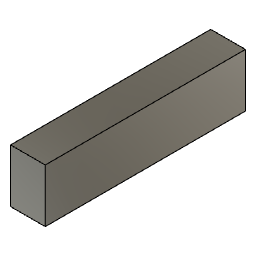
스위치 홈 (Autodesk Fusion 360 design; units mm, degrees)
Autodesk Fusion 360 part; units mm, degrees
note: some values were not read from the file. Set by a fixed rule: which face or edge a step refers to.
sketch "스케치1" plane through (0, 0, 0) normal (0, 0, 1) x (1, 0, 0)
  line L0 (-5, 0) -> (15, 0)
  line L1 (15, 0) -> (15, -30)
  line L2 (15, -30) -> (-5, -30)
  line L3 (-5, -30) -> (-5, 0)
  line L4 (-5, 0) -> (15, 0)
  line L5 (15, 0) -> (15, 50)
  line L6 (15, 50) -> (-5, 50)
  line L7 (-5, 50) -> (-5, 0)
  line L8 (-4, 50) -> (-4, 45)
  line L9 (-4, 45) -> (-4, 0)
  line L10 (14, 50) -> (14, 0)
  line L11 (-5, -30) -> (-5, 0)
  line L12 (15, 0) -> (15, -30)
  line L13 (15, -30) -> (-5, -30)
  line L14 (15, 50) -> (-5, 50)
  line L15 (-5, 0) -> (15, 0)
  line L16 (14, 50) -> (14, 0)
  line L17 (15, 0) -> (15, 50)
  line L18 (-5, 0) -> (15, 0)
  line L19 (-5, 50) -> (-5, 0)
  line L20 (-5, 0) -> (-5, 30)
  line L21 (15, 30) -> (-5, 30)
  line L22 (-5, 0) -> (-5, 40)
  line L23 (-5, 40) -> (15, 40)
  line L24 (-5, -10) -> (15, -10)
  line L25 (125, 0) -> (125, 30)
  line L26 (125, 0) -> (125, 40)
  line L27 (125, 40) -> (145, 40)
  line L28 (125, 50) -> (125, 0)
  line L29 (125, -10) -> (145, -10)
  line L30 (145, 0) -> (145, -30)
  line L31 (144, 50) -> (144, 0)
  line L32 (126, 45) -> (126, 0)
  line L33 (144, 50) -> (144, 0)
  line L34 (125, -30) -> (125, 0)
  line L35 (145, 50) -> (125, 50)
  line L36 (145, -30) -> (125, -30)
  line L37 (125, -30) -> (125, 0)
  line L38 (125, 0) -> (145, 0)
  line L39 (125, 0) -> (145, 0)
  line L40 (145, -30) -> (125, -30)
  line L41 (125, 0) -> (145, 0)
  line L42 (145, 0) -> (145, -30)
  line L43 (145, 30) -> (125, 30)
  line L44 (125, 0) -> (145, 0)
  line L45 (145, 0) -> (145, 50)
  line L46 (125, 50) -> (125, 0)
  line L47 (145, 50) -> (125, 50)
  line L48 (145, 0) -> (145, 50)
  line L49 (126, 50) -> (126, 45)
  point P0 (130, 0)
  point P1 (130, 0)
  dimension "d1" = 30
  dimension "d2" = 20
  dimension "d3" = 50
  dimension "d6" = 1
  dimension "d7" = 1
  dimension "d8" = 30
  dimension "d9" = 20
  dimension "d10" = 50
  dimension "d12" = 1
  dimension "d23" = 30
  dimension "d24" = 40
  dimension "d25" = 10
  dimension "d26" = 30
  dimension "d27" = 20
  dimension "d28" = 50
  dimension "d29" = 1
  dimension "d30" = 1
  dimension "d31" = 30
  dimension "d32" = 20
  dimension "d33" = 50
  dimension "d34" = 1
  dimension "d35" = 30
  dimension "d36" = 40
  dimension "d37" = 10
  constraint horizontal L0
  constraint vertical L1
  constraint horizontal L2
  constraint vertical L3
  constraint horizontal L4
  constraint vertical L5
  constraint horizontal L6
  constraint vertical L7
  constraint coincident L6 L8.start
  constraint perpendicular L6 L8
  constraint coincident L0 L9.end
  constraint perpendicular L0 L9
  constraint coincident L6 L10.start
  constraint coincident L0 L10.end
  constraint perpendicular L6 L10
  constraint horizontal L15
  constraint vertical L12
  constraint horizontal L13
  constraint vertical L11
  constraint horizontal L18
  constraint vertical L17
  constraint horizontal L14
  constraint vertical L19
  constraint coincident L10.start L14
  constraint coincident L10.end L15
  constraint perpendicular L14 L16
  constraint coincident L19 L20.end
  constraint perpendicular L4 L20
  constraint coincident L5 L21.start
  constraint perpendicular L7 L21
  constraint perpendicular L21 L22
  constraint coincident L17 L23.end
  constraint perpendicular L17 L23
  constraint coincident L1 L24.end
  constraint perpendicular L1 L24
  constraint horizontal L41
  constraint vertical L42
  constraint horizontal L36
  constraint vertical L34
  constraint horizontal L38
  constraint vertical L48
  constraint horizontal L47
  constraint vertical L28
  constraint coincident L49.start L47
  constraint perpendicular L47 L49
  constraint coincident L32.end L41
  constraint perpendicular L32 L41
  constraint coincident L31.start L47
  constraint coincident L31.end L41
  constraint perpendicular L31 L47
  constraint horizontal L44
  constraint vertical L30
  constraint horizontal L40
  constraint vertical L37
  constraint horizontal L39
  constraint vertical L45
  constraint horizontal L35
  constraint vertical L46
  constraint coincident L31.start L35
  constraint coincident L31.end L44
  constraint perpendicular L33 L35
  constraint coincident L25.end L46
  constraint perpendicular L25 L38
  constraint coincident L43.start L48
  constraint perpendicular L28 L43
  constraint perpendicular L26 L43
  constraint coincident L27.end L45
  constraint perpendicular L27 L45
  constraint coincident L29.end L42
  constraint perpendicular L29 L42
  measures "d1" distance of L0.end L1.end
  measures "d2" distance of L1.end L2.end
  measures "d3" distance of L0.end L5.end
  measures "d6" distance of L7 L9
  measures "d7" distance of L5 L10
  measures "d8" distance of L0.end L1.end
  measures "d9" distance of L1.end L2.end
  measures "d10" distance of L5.end L0.end
  measures "d12" distance of L16 L17
  measures "d23" distance of L15 L21
  measures "d24" distance of L0.start L22.end
  measures "d25" distance of L0.start L24.start
  measures "d26" distance of L30.start L30.end
  measures "d27" distance of L30.end L34.start
  measures "d28" distance of L35.start L30.start
  measures "d29" distance of L28 L32
  measures "d30" distance of L31 L48
  measures "d31" distance of L30.end L30.start
  measures "d32" distance of L34.start L30.end
  measures "d33" distance of L30.start L35.start
  measures "d34" distance of L33 L45
  measures "d35" distance of L43 L44
  measures "d36" distance of L25.start L26.end
  measures "d37" distance of L25.start L29.start
extrude "돌출1" add sketch "스케치1" along normal blind 30 contours L1 L2 L3 L11 L12 L13 L24 makes body 1
extrude "돌출2" add sketch "스케치1" along normal blind 30 contours L0 L1 L3 L4 L11 L12 L15 L18 L24 bodies 1
extrude "돌출3" add sketch "스케치1" along normal blind 30 contours L0 L4 L5 L10 L15 L16 L17 L18 L21 bodies 1
extrude "돌출4" add sketch "스케치1" along normal blind 30 contours L0 L4 L7 L9 L15 L18 L19 L20 L21 L22 bodies 1
extrude "돌출5" add sketch "스케치1" along normal blind 30 separate body contours L29 L30 L34 L36 L37 L40 L42 makes body 2
extrude "돌출6" add sketch "스케치1" along normal blind 30 contours L29 L30 L34 L37 L38 L39 L41 L42 L44 bodies 2
extrude "돌출7" add sketch "스케치1" along normal blind 30 contours L25 L26 L28 L32 L38 L39 L41 L43 L44 L46 | L31 L33 L38 L39 L41 L43 L44 L45 L48 bodies 2
extrude "돌출8" add sketch "스케치1" along normal blind 30 contours L7 L9 L19 L21 L22 L23 | L6 L7 L8 L9 L14 L19 L23 | L5 L10 L16 L17 L21 L23 | L5 L6 L10 L14 L16 L17 L23 | L26 L27 L28 L32 L43 L46 | L27 L28 L32 L35 L46 L47 L49 | L27 L31 L33 L43 L45 L48 | L27 L31 L33 L35 L45 L47 L48 bodies 1 2
extrude "돌출9" cut 2 faces at (138, -20, 30) (8, -20, 30) along direction (0, 0, -1) blind 10 on bodies 1 2 bodies 1 2
sketch "스케치2" plane through (0, 0, 0) normal (0, 1, 0) x (-1, 0, 0)
  line L0 (4, 20) -> (-14, 20)
  line L1 (-14, 20) -> (-14, 0)
  line L2 (-14, 0) -> (4, 0)
  line L3 (4, 0) -> (4, 20)
  line L4 (-126, 20) -> (-144, 20)
  line L5 (-144, 20) -> (-144, 0)
  line L6 (-144, 0) -> (-126, 0)
  line L7 (-126, 0) -> (-126, 20)
  line L8 (-138, 17) -> (-128, 17)
  line L9 (-128, 17) -> (-128, 3)
  line L10 (-128, 3) -> (-138, 3)
  line L11 (-138, 3) -> (-138, 17)
  line L12 (-12, 17) -> (-2, 17)
  line L13 (-2, 17) -> (-2, 3)
  line L14 (-2, 3) -> (-12, 3)
  line L15 (-12, 3) -> (-12, 17)
  dimension "d56" = 2
  dimension "d57" = 2
  dimension "d58" = 10
  dimension "d59" = 10
  constraint horizontal L8
  constraint vertical L9
  constraint horizontal L10
  constraint vertical L11
  constraint horizontal L12
  constraint vertical L13
  constraint horizontal L14
  constraint vertical L15
  measures "d56" distance of L7 L9
  measures "d57" distance of L1 L15
  measures "d58" distance of L9 L11
  measures "d59" distance of L13 L15
extrude "돌출10" cut sketch "스케치2" against normal blind 10 contours L8 L9 L10 L11 | L12 L13 L14 L15 bodies 1 2
extrude "돌출11" cut 2 faces at (131.3333, -10, 7.6667) (8.6667, -10, 12.3333) along direction (0, -1, 0) blind 15 on bodies 1 2 bodies 1 2
extrude "돌출12" add sketch "스케치1" along normal blind 20 contours L27 L31 L32 L33 L35 L47 L49 bodies 2
extrude "돌출13" cut 1 faces at (131.3333, -25, 7.6667) along direction (0, 1, 0) blind 75 on bodies 2 bodies 2
move_face "면 간격띄우기1" offset -2 2 faces at (134.6667, 43.3333, 17) (131.3333, 43.3333, 3) on bodies 2
extrude "돌출14" add 1 faces at (134.6667, -25, 12.3333) along direction (0, 1, 0) blind 25 on bodies 2 bodies 2
extrude "돌출15" add sketch "스케치1" along normal blind 20 contours L6 L8 L9 L10 L14 L16 L23 bodies 1
move_face "면 간격띄우기2" offset -4 1 faces at (2, -8.3333, 12.3333) on bodies 1
sketch "스케치3" plane through (0, 0, 20) normal (0, 0, 1) x (-1, 0, 0)
  line L0 (-14, -40) -> (-14, 0)
  line L1 (-14, 0) -> (4, 0)
  line L2 (4, 0) -> (4, -40)
  line L3 (4, -40) -> (-14, -40)
  line L4 (-15, -50) -> (5, -50)
  line L5 (5, -50) -> (5, 30)
  line L6 (5, 30) -> (-15, 30)
  line L7 (-15, 30) -> (-15, -50)
  line L8 (-14, 26.9594) -> (4, 26.9594)
  line L9 (4, 26.9594) -> (4, 21.9594)
  line L10 (4, 21.9594) -> (-14, 21.9594)
  line L11 (-14, 21.9594) -> (-14, 26.9594)
  dimension "d74" = 5
  constraint horizontal L8
  constraint vertical L9
  constraint horizontal L10
  constraint vertical L11
  measures "d74" distance of L8.start L10.end
extrude "돌출16" cut sketch "스케치3" against normal blind 18 contours L8 L9 L10 L11 bodies 1
extrude "돌출17" add 1 faces at (8, -25.2927, 2) along direction (0, 0, 1) blind 1 on bodies 1 bodies 1
move_face "면 간격띄우기3" offset 5 1 faces at (138, 46.6667, 7) on bodies 2
move_face "면 간격띄우기4" offset 2 2 faces at (12, -7.3198, 7.6667) (-2, -7.3198, 12.3333) on bodies 1
extrude "돌출18" add sketch "스케치1" along normal blind 2 from surface at 18 contours L0 L4 L9 L10 L15 L16 L18 L21 | L9 L10 L16 L21 L23 bodies 1
extrude "돌출19" add sketch "스케치1" along normal blind 3 from surface at 17 contours L31 L32 L33 L38 L39 L41 L43 L44 | L27 L31 L32 L33 L43 bodies 2
extrude "돌출20" add sketch "스케치1" against normal blind 1 from surface at 17 separate body contours L0 L4 L9 L10 L15 L16 L18 L21 | L9 L10 L16 L21 L23 makes body 3
extrude "돌출21" add 1 faces at (134.3333, 13.3333, 17) along direction (0, 0, -1) blind 1 on bodies 2 bodies 2
extrude "돌출22" add 1 faces at (131.3333, 43.3333, 19) along direction (0, 0, -1) blind 1 on bodies 2 bodies 2
extrude "돌출23" add 1 faces at (131.3333, 43.3333, 18) along direction (0, 0, -1) blind 1 on bodies 2 bodies 2
move_face "면 간격띄우기5" offset -1 1 faces at (131.3333, 43.3333, 17) on bodies 2
move_face "면 간격띄우기6" offset 8 1 faces at (144, 26.6667, 10.6667) on bodies 2
move_face "면 간격띄우기7" offset -7 1 faces at (145, 23.3333, 6.6667) on bodies 2
move_face "면 간격띄우기8" offset 5 1 faces at (0, -14.6396, 7.6667) on bodies 1
move_face "면 간격띄우기9" offset 8 1 faces at (-4, 13.3333, 12) on bodies 1
move_face "면 간격띄우기10" offset -7 1 faces at (-5, -3.3333, 13.3333) on bodies 1
extrude "돌출24" cut 2 faces at (-4, 20, 16.3333) (-4, 36.6667, 16.3333) along direction (1, 0, 0) blind 6 on bodies 3 bodies 3
combine "결합1" operation add target body 3 tool bodies 1
move_face "면 간격띄우기11" offset 2 1 faces at (131.3333, 46.6667, 1) on bodies 2
extrude "돌출25" cut 1 faces at (136.3333, 50, 7.6667) along direction (0, -1, 0) blind 5 on bodies 2 bodies 2
move_face "면 간격띄우기12" offset -2 1 faces at (133, 43.3333, 12.3333) on bodies 2
move_face "면 간격띄우기13" offset -1 2 faces at (132.6667, 43.3333, 3) (130.3333, 43.3333, 18) on bodies 2
move_face "면 간격띄우기14" offset 0.5 1 faces at (126, 26.6667, 10.6667) on bodies 2
move_face "면 간격띄우기15" offset -0.5 1 faces at (136, 26.6667, 10.6667) on bodies 2
hidden bodies 3
